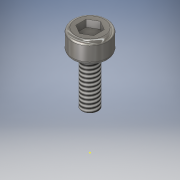
# Autodesk Inventor part: screw
Saved by Autodesk Inventor 2016 (Build 200138000, 138)
## iProperties
Created: 2015-05-11
Part Number: screw
Material: Generic
Document SubType Name: Modeling
Designer: Admin
Density: 1 g/cm^3
Appearance: Default
Mass: 0.0811184 g
Surface Area: 1.38953 cm^2
Volume: 0.0811184 cm^3
Author: Admin
Autodesk Inventor part; units mm, degrees
ref_plane "YZ Plane" through (0, 0, 0) normal (1, 0, 0) x (0, 1, 0)
ref_plane "XZ Plane" through (0, 0, 0) normal (0, 1, 0) x (-1, 0, 0)
ref_plane "XY Plane" through (0, 0, 0) normal (0, 0, 1) x (1, 0, 0)
sketch "Sketch1" plane through (0, 0, 0) normal (0, 1, 0) x (-1, 0, 0)
  circle A0 centre (0, 0) radius 1.143
  dimension "d24" = 2.286
  constraints: 1 centre point
  measures "d24" diameter of A0
extrude "Extrusion1" add sketch "Sketch1" along normal blind 12.5
sketch "Sketch2" plane through (0, 12.5, 0) normal (0, 1, 0) x (1, 0, 0)
  circle A0 centre (0, 0) radius 1.5 projected
  circle A1 centre (0, 0) radius 2.54
  dimension "d3" = 5.08
  constraints: 1 centre point, 1 coincident
  measures "d3" diameter of A1
extrude "Extrusion2" add sketch "Sketch2" along normal blind 3 contours A0 | A1
fillet "Fillet1" radius 0.508 2 edges at (-2.54, 15.5, 0) (-2.54, 12.5, 0)
sketch "Sketch3" plane through (0, 15.5, 0) normal (0, 1, 0) x (1, 0, 0)
  line L0 (0, 0) -> (1.5, 0) construction
  line L1 (-1.299, -0.75) -> (-1.299, 0.75)
  line L2 (-1.299, 0.75) -> (0.0002, 1.5)
  line L3 (1.299, 0.75) -> (0.0002, 1.5)
  line L4 (1.299, 0.75) -> (1.299, -0.75)
  line L5 (0, -1.5) -> (1.299, -0.75)
  line L6 (-1.299, -0.75) -> (0, -1.5)
  constraints: 14 end point, 1 horizontal
extrude "Extrusion4" cut sketch "Sketch3" against normal blind 1
sketch "Sketch4" plane through (0, 0, 0) normal (0, 0, 1) x (1, 0, 0)
  point P0 (0, 0)
sketch "Sketch5" plane through (0, 0, 0) normal (0, -1, 0) x (1, 0, 0)
  circle A0 centre (0, 0) radius 3.3551
  constraints: 1 centre point, 1 coincident
extrude "Extrusion5" cut sketch "Sketch5" against normal blind 5.715
thread "Thread3" size "3-48 UNC" class "2A" standard "ANSI Unified Screw Threads" full length
body "Solid1"
